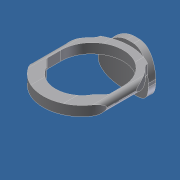
# Autodesk Inventor part: HFC12_Thumb_Latch.
Saved by Autodesk Inventor 2012 SP1 (Build 160190100, 190)
## iProperties
Category: PARTsolutions
Created: 2012-06-06
Part Number: HFC12_Thumb_Latch.
Catalog Web Link: www.cadenas.de
Description: HFC12 Thumb Latch - HFC12 Thumb Latch
Document SubType Name: Modeling
Designer: PARTsolutions
Material: Default
Mass: 1.83094 g
Surface Area: 19.9101 cm^2
Volume: 1.83094 cm^3
Density: 1 g/cm^3
NB: HFC12_Thumb_Latch.
NN: HFC12 Thumb Latch
NT: HFC12 Thumb Latch
NBSYN: $PN..
LINA: HFC12_Thumb_Latch.
PN: HFC12_Thumb_Latch
KT: DUMMY
SUPPLIER: Colder
ARTICLENO: HFC12_Thumb_Latch.HI
BOMINFO: HFC12_Thumb_Latch.
CREATOR: CADENAS GmbH
PSOL_IDENT_0: {\\10.0.0.251\data_v9\23d-libs\colder\single_line\3_8_nom_flow\hfc12_series\bodies\parts\hfc12_thumb
PSOL_IDENT_1: _latch.prj},189 {VTYP=3D},{NB=HFC12_Thumb_Latch.},{LINA=HFC12_Thumb_Latch.},{NN=HFC12 Thumb Latch},{
PSOL_IDENT_2: DATE=12.11.2009 08:26:07},{GEOMDATE=12.11.2009 08:26:00},{VERSION=},{LINEID=10},{LINESUBID=-1},{WBVA
PSOL_IDENT_3: R=}  {NB=HFC12_Thumb_Latch.},{LINA=HFC12_Thumb_Latch.},{KT=DUMMY},{PN=HFC12_Thumb_Latch}
Title: HFC12_Thumb_Latch.
Author: Cadenas PARTsolutions
Comments: HFC12 Thumb Latch
Autodesk Inventor part; units mm, degrees
sketch "Sketch1" plane through (0, 0, 31.624) normal (0, 0, 1) x (1, 0, 0)
  arc A0 (9.9059, 15.9738) -> (-9.9059, 15.9738) centre (0, 0) ccw
  line L0 (9.9059, 15.9738) -> (9.9059, 18.8971)
  arc A1 (9.9059, 18.8971) -> (-9.9059, 18.8971) centre (0, 0) ccw
  line L1 (-9.9059, 18.8971) -> (-9.9059, 15.9738)
  constraints: 4 end point, 4 point on circle, 2 centre point
extrude "Extrusion1" add sketch "Sketch1" along normal mid plane 17.3715
sketch "Sketch4" plane through (0, 0, 0) normal (0, 1, 0) x (-1, 0, 0)
  line L0 (21.7076, 15.4624) -> (21.7076, 45.6279)
  line L1 (21.7076, 45.6279) -> (-19.8126, 45.6279)
  line L2 (-19.8126, 45.6279) -> (-19.8126, 15.4624)
  line L3 (-19.8126, 15.4624) -> (21.7076, 15.4624)
  arc A0 (1.1925, 23.0378) -> (1.1925, 40.3098) centre (1.1925, 31.6738) ccw
  line L4 (1.1925, 40.3098) -> (-1.2025, 40.3098)
  arc A1 (-1.2025, 40.3098) -> (-1.3475, 23.0378) centre (-1.2944, 31.674) ccw
  line L5 (-1.3475, 23.0378) -> (1.1925, 23.0378)
  constraints: 12 end point, 4 point on circle, 2 centre point
extrude "Extrusion2" cut sketch "Sketch4" along normal blind 21.3026
sketch "Sketch7" plane through (0, 0, 36.7659) normal (0, 0, 1) x (1, 0, 0)
  line L0 (-14.603, 0) -> (-14.603, -1.2396)
  line L1 (-14.603, -1.2396) -> (-14.478, -1.7062)
  line L2 (-14.478, -1.7062) -> (-14.4779, -4.6768)
  arc A0 (-14.4779, -4.6768) -> (-14.4517, -4.8381) centre (-13.9698, -4.6768) ccw
  arc A1 (-14.4517, -4.8381) -> (14.4517, -4.8381) centre (0, 0) ccw
  arc A2 (14.4517, -4.8381) -> (14.4779, -4.6767) centre (13.969, -4.6767) ccw
  line L3 (14.4779, -4.6767) -> (14.478, -1.7062)
  line L4 (14.478, -1.7062) -> (14.603, -1.2396)
  line L5 (14.603, -1.2396) -> (14.603, 0)
  line L6 (14.603, 0) -> (14.478, 0)
  line L7 (14.478, 0) -> (14.478, 6.5848)
  arc A3 (14.478, 6.5848) -> (10.0998, 14.5858) centre (0, 3.8608) ccw
  arc A4 (9.3033, 16.3321) -> (10.0998, 14.5858) centre (11.8412, 16.4349) ccw
  arc A5 (9.3033, 16.3321) -> (-9.3033, 16.3321) centre (0, 0) ccw
  arc A6 (-10.0998, 14.5858) -> (-9.3033, 16.3321) centre (-11.8412, 16.4349) ccw
  arc A7 (-10.0998, 14.5858) -> (-14.478, 6.5848) centre (0, 3.8608) ccw
  line L8 (-14.478, 6.5848) -> (-14.478, 0)
  line L9 (-14.478, 0) -> (-14.603, 0)
  line L10 (-12.192, 3.8608) -> (-12.192, -1.2519)
  arc A8 (-12.192, -1.2519) -> (-11.82, -2.15) centre (-10.922, -1.2519) ccw
  line L11 (-11.82, -2.15) -> (-9.3148, -4.6552)
  arc A9 (-9.3148, -4.6552) -> (9.3148, -4.6552) centre (0, 0) ccw
  line L12 (9.3148, -4.6552) -> (11.82, -2.15)
  arc A10 (11.82, -2.15) -> (12.192, -1.2519) centre (10.922, -1.2519) ccw
  line L13 (12.192, -1.2519) -> (12.192, 3.8608)
  arc A11 (12.192, 3.8608) -> (6.858, 13.9411) centre (0, 3.8608) ccw
  arc A12 (6.858, 13.9411) -> (-6.858, 13.9411) centre (0, 3.8608) ccw
  arc A13 (-6.858, 13.9411) -> (-12.192, 3.8608) centre (0, 3.8608) ccw
  constraints: 28 end point, 28 point on circle, 14 centre point
extrude "Extrusion3" add sketch "Sketch7" along normal mid plane 3.8347
sketch "Sketch_2" plane through (0, 0, 0) normal (0, 1, 0) x (-1, 0, 0)
  line L0 (21.7076, 15.4624) -> (21.7076, 45.6279)
  line L1 (21.7076, 45.6279) -> (-19.8126, 45.6279)
  line L2 (-19.8126, 45.6279) -> (-19.8126, 15.4624)
  line L3 (-19.8126, 15.4624) -> (21.7076, 15.4624)
  arc A0 (13.0066, 34.8988) -> (12.573, 38.6588) centre (12.573, 36.7538) ccw
  line L4 (12.573, 38.6588) -> (6.2709, 38.6588)
  arc A1 (6.2709, 38.6588) -> (1.1925, 40.3098) centre (1.1925, 31.6738) ccw
  line L5 (1.1925, 40.3098) -> (-1.3675, 40.3098)
  arc A2 (-1.3675, 40.3098) -> (-6.3931, 38.6588) centre (-1.3144, 31.674) ccw
  line L6 (-6.3931, 38.6588) -> (-12.573, 38.6588)
  arc A3 (-12.573, 38.6588) -> (-13.0066, 34.8988) centre (-12.573, 36.7538) ccw
  line L7 (-13.0066, 34.8988) -> (-9.3061, 34.8988)
  arc A4 (-9.3061, 34.8988) -> (-1.3475, 23.0378) centre (-1.2944, 31.674) ccw
  line L8 (-1.3475, 23.0378) -> (1.1925, 23.0378)
  arc A5 (1.1925, 23.0378) -> (9.2037, 34.8988) centre (1.1925, 31.6738) ccw
  line L9 (9.2037, 34.8988) -> (13.0066, 34.8988)
  constraints: 20 end point, 12 point on circle, 6 centre point
extrude "Extrusion4" cut sketch "Sketch_2" along normal mid plane 42.5868
sketch "Sketch13" plane through (0, 19, 0) normal (0, 1, 0) x (-1, 0, 0)
  arc A0 (-2.0647, 31.2687) -> (-1.8483, 30.1905) centre (-1.8321, 30.7546) ccw
  line L0 (-1.8483, 30.1905) -> (1.6098, 30.4859)
  line L1 (1.6098, 30.4859) -> (2.3072, 31.8095)
  line L2 (2.3072, 31.8095) -> (5.4582, 32.4022)
  line L3 (5.4582, 32.4022) -> (6.754, 32.5229)
  line L4 (6.754, 32.5229) -> (7.4361, 32.5229)
  arc A1 (7.6125, 31.7185) -> (7.4361, 32.5229) centre (7.4361, 32.1013) ccw
  line L5 (7.6125, 31.7185) -> (6.7015, 31.3927)
  line L6 (6.7015, 31.3927) -> (5.3534, 31.0166)
  line L7 (5.3534, 31.0166) -> (4.8016, 30.9039)
  line L8 (4.8016, 30.9039) -> (4.216, 30.8237)
  arc A2 (4.216, 30.8237) -> (4.272, 30.2037) centre (4.2298, 30.5124) ccw
  line L9 (4.272, 30.2037) -> (4.9596, 30.2978)
  line L10 (4.9596, 30.2978) -> (5.5116, 30.4105)
  line L11 (5.5116, 30.4105) -> (6.9652, 30.8162)
  line L12 (6.9652, 30.8162) -> (7.8754, 31.1416)
  arc A3 (7.8754, 31.1416) -> (7.4361, 33.1449) centre (7.4361, 32.0951) ccw
  line L13 (7.4361, 33.1449) -> (6.7552, 33.1449)
  line L14 (6.7552, 33.1449) -> (5.312, 33.0107)
  line L15 (5.312, 33.0107) -> (2.6792, 32.5154)
  line L16 (2.6792, 32.5154) -> (3.0109, 33.1449)
  line L17 (3.0109, 33.1449) -> (2.2353, 33.1449)
  line L18 (2.2353, 33.1449) -> (1.8183, 32.3535)
  line L19 (1.8183, 32.3535) -> (1.1846, 32.2343)
  line L20 (1.1846, 32.2343) -> (-1.07, 31.6244)
  line L21 (-1.07, 31.6244) -> (-2.0647, 31.2687)
  line L22 (-1.4814, 30.8064) -> (1.1204, 31.029)
  line L23 (1.1204, 31.029) -> (1.4463, 31.6476)
  line L24 (1.4463, 31.6476) -> (1.3307, 31.6259)
  line L25 (1.3307, 31.6259) -> (-0.8077, 31.0473)
  line L26 (-0.8077, 31.0473) -> (-1.4814, 30.8064)
  constraints: 54 end point, 8 point on circle, 4 centre point
extrude "Extrusion5" cut sketch "Sketch13" along normal blind 3
sketch "Sketch16" plane through (0, 19, 0) normal (0, 1, 0) x (-1, 0, 0)
  arc A0 (-8.3321, 32.5762) -> (-8.1861, 31.9677) centre (-8.244, 32.2756) ccw
  line L0 (-8.1861, 31.9677) -> (-5.8757, 32.4023)
  line L1 (-5.8757, 32.4023) -> (-4.5792, 32.5229)
  line L2 (-4.5792, 32.5229) -> (-3.4543, 32.5229)
  arc A1 (-3.2794, 31.7265) -> (-3.4543, 32.5229) centre (-3.4543, 32.1055) ccw
  line L3 (-3.2794, 31.7265) -> (-4.0387, 31.455)
  line L4 (-4.0387, 31.455) -> (-5.6997, 31.0055)
  line L5 (-5.6997, 31.0055) -> (-6.3105, 30.8906)
  arc A2 (-6.8282, 30.8237) -> (-6.3105, 30.8906) centre (-7.1494, 35.3504) ccw
  arc A3 (-6.8282, 30.8237) -> (-6.772, 30.2037) centre (-6.794, 30.5143) ccw
  arc A4 (-6.772, 30.2037) -> (-6.1642, 30.2821) centre (-7.149, 35.5175) ccw
  line L6 (-6.1642, 30.2821) -> (-5.5552, 30.3967)
  line L7 (-5.5552, 30.3967) -> (-3.7744, 30.8786)
  line L8 (-3.7744, 30.8786) -> (-3.0161, 31.1497)
  arc A5 (-3.0161, 31.1497) -> (-3.4543, 33.1449) centre (-3.3627, 32.1193) ccw
  line L9 (-3.4543, 33.1449) -> (-4.5788, 33.1449)
  line L10 (-4.5788, 33.1449) -> (-6.0223, 33.0107)
  line L11 (-6.0223, 33.0107) -> (-8.3321, 32.5762)
  constraints: 24 end point, 12 point on circle, 6 centre point
extrude "Extrusion6" cut sketch "Sketch16" along normal blind 3
ref_plane "0_XY" through (0, 0, 0) normal (0, 0, 1) x (1, 0, 0)
ref_plane "0_YZ" through (0, 0, 0) normal (1, 0, 0) x (0, 1, 0)
ref_plane "0_ZX" through (0, 0, 0) normal (0, 1, 0) x (0, 0, 1)
body "Solid1"
